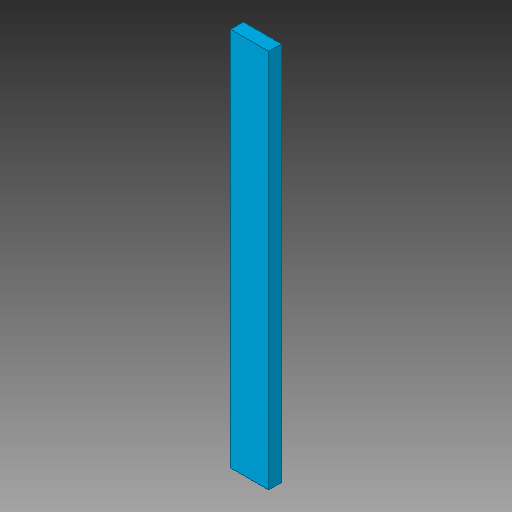
# Autodesk Inventor part: Pieza Prueba
Saved by Autodesk Inventor 2018 (Build 220112000, 112)
## iProperties
Created: 2019-05-20
Part Number: Pieza Prueba
Material: Generic
Document SubType Name: Modeling
Designer: Ivan
Density: 1 g/cm^3
Appearance: Default
Mass: 5.76 g
Surface Area: 39.36 cm^2
Volume: 5.76 cm^3
Author: Ivan
Autodesk Inventor part; units mm, degrees
ref_plane "YZ Plane" through (0, 0, 0) normal (1, 0, 0) x (0, 1, 0)
ref_plane "XZ Plane" through (0, 0, 0) normal (0, 1, 0) x (-1, 0, 0)
ref_plane "XY Plane" through (0, 0, 0) normal (0, 0, 1) x (1, 0, 0)
sketch "Sketch1" plane through (0, 0, 0) normal (0, 0, 1) x (1, 0, 0)
  line L0 (-6, 60) -> (6, 60)
  line L1 (6, 60) -> (6, -60)
  line L2 (6, -60) -> (-6, -60)
  line L3 (-6, -60) -> (-6, 60)
  point P0 (0, 0)
  point P1 (0, 60)
  point P2 (6, 0)
  dimension "d0" = 120
  dimension "d1" = 12
  constraints: 8 end point, 2 midpoint, 2 parallel, 1 horizontal, 1 horizontal alignment, 1 perpendicular, 1 vertical alignment
  measures "d0" distance of L0.end L1.end
  measures "d1" distance between parallel lines of L3 L1
extrude "Extrusion1" add sketch "Sketch1" along normal blind 4
body "Solid1"
